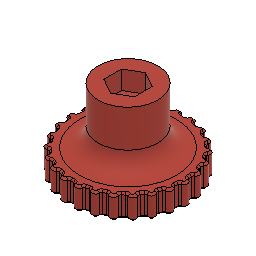
04 Laser Focus Knob v1 (Autodesk Fusion 360 design; units mm, degrees)
Autodesk Fusion 360 part; units mm, degrees
note: some values were not read from the file. Set by a fixed rule: which sketch regions a step uses.
sketch "Sketch1" plane through (0, 0, 0) normal (0, 1, 0) x (1, 0, 0)
  circle A0 centre (0, 0) radius 15
  dimension "d1" = 30
  constraint coincident A0.centre origin
  measures "d1" diameter of A0
extrude "Extrude1" add sketch "Sketch1" along normal blind 6
sketch "Sketch2" plane through (0, 6, 0) normal (0, 1, 0) x (-1, 0, 0)
  circle A0 centre (0, 0) radius 15
  circle A1 centre (0, 0) radius 8
  dimension "d4" = 16
  constraint concentric A0 A1
  measures "d4" diameter of A1
extrude "Extrude2" add sketch "Sketch2" along normal blind 15 contours A1
sketch "Sketch3" plane through (0, 21, 0) normal (0, 1, 0) x (-1, 0, 0)
  circle A0 centre (0, 0) radius 8
  circle A1 centre (0, 0) radius 2.625
  dimension "d7" = 5.25
  constraint concentric A0 A1
  measures "d7" diameter of A1
extrude "Extrude3" cut sketch "Sketch3" against normal blind 50 contours A1
sketch "Sketch4" plane through (0, 0, 0) normal (0, -1, 0) x (1, 0, 0)
  circle A0 centre (0, 0) radius 2.625
  circle A1 centre (0, 0) radius 15
  circle A2 centre (0, 0) radius 5
  dimension "d10" = 10
  constraint concentric A0 A2
  measures "d10" diameter of A2
extrude "Extrude4" cut sketch "Sketch4" against normal blind 12 contours A2
sketch "Sketch5" plane through (0, 21, 0) normal (0, 1, 0) x (-1, 0, 0)
  circle A0 centre (0, 0) radius 2.625
  circle A1 centre (0, 0) radius 8
  line L0 (-4.1, -2.3671) -> (0, -4.7343)
  line L1 (0, -4.7343) -> (4.1, -2.3671)
  line L2 (4.1, -2.3671) -> (4.1, 2.3671)
  line L3 (4.1, 2.3671) -> (0, 4.7343)
  line L4 (0, 4.7343) -> (-4.1, 2.3671)
  line L5 (-4.1, 2.3671) -> (-4.1, -2.3671)
  dimension "d27" = 8.2
  constraint coincident A0.centre A1.centre
  measures "d27" distance of L2 L5
extrude "Extrude5" cut sketch "Sketch5" against normal blind 5 contours L0 L1 L2 L3 L4 L5
sketch "Sketch6" plane through (0, 0, 0) normal (0, -1, 0) x (1, 0, 0)
  circle A0 centre (0, 0) radius 5
  circle A1 centre (0, 0) radius 15
  circle A2 centre (-15, 0) radius 1
  point P0 (-15, 0)
  dimension "d15" = 2
  constraint coincident P0 A2.centre
  measures "d15" diameter of A2
extrude "Extrude6" add sketch "Sketch6" against normal blind 6 contours A1 A2 | A1 A2 picked at (-14.6642, 0) picked at (-15.3309, 0)
fillet "Fillet1" radius 0.5 1 edges at (-14.9667, 3, 0.9994)
fillet "Fillet2" radius 0.5 1 edges at (-14.9667, 3, -0.9994)
pattern_circular "C-Pattern1" count 26 over 360 about axis through (0, 1.75, 0) along (0, 1, 0) of "Extrude6", "Fillet1", "Fillet2"
chamfer "Chamfer1" distance 0.5 angle 45 208 edges at (-9.089, 0, 13.1677) (-9.4686, 0, 11.7468) (-9.9468, 0, 11.2277) (-10.5198, 0, 10.8155) (-11.9762, 0, 10.61) (-12.0047, 0, 9.1394) (-12.3448, 0, 8.521) (-12.8024, 0, 7.9837) (-14.1673, 0, 7.4356) (-13.8431, 0, 6.001) (-14.0252, 0, 5.3191) (-14.341, 0, 4.6879) (-15.5351, 0, 3.8291) (-14.8769, 0, 2.5137) (-14.8906, 0, 1.8081) (-15.0462, 0, 1.1196) (-16, 0, 0) (-15.0462, 0, -1.1196) (-14.8906, 0, -1.8081) (-14.8769, 0, -2.5137) (-15.5351, 0, -3.8291) (-14.341, 0, -4.6879) (-14.0252, 0, -5.3191) (-13.8431, 0, -6.001) (-14.1673, 0, -7.4356) (-12.8024, 0, -7.9837) (-12.3448, 0, -8.521) (-12.0047, 0, -9.1394) (-11.9762, 0, -10.61) (-10.5198, 0, -10.8155) (-9.9468, 0, -11.2277) (-9.4686, 0, -11.7468) (-9.089, 0, -13.1677) (-7.6258, 0, -13.0188) (-6.9708, 0, -13.2818) (-6.3823, 0, -13.6714) (-5.6737, 0, -14.9603) (-4.2886, 0, -14.4655) (-3.5897, 0, -14.5641) (-2.9251, 0, -14.8015) (-1.9286, 0, -15.8833) (-0.7022, 0, -15.0715) (0, 0, -15) (0.7022, 0, -15.0715) (1.9286, 0, -15.8833) (2.9251, 0, -14.8015) (3.5897, 0, -14.5641) (4.2886, 0, -14.4655) (5.6737, 0, -14.9603) (6.3823, 0, -13.6714) (6.9708, 0, -13.2818) (7.6258, 0, -13.0188) (9.089, 0, -13.1677) (9.4686, 0, -11.7468) (9.9468, 0, -11.2277) (10.5198, 0, -10.8155) (11.9762, 0, -10.61) (12.0047, 0, -9.1394) (12.3448, 0, -8.521) (12.8024, 0, -7.9837) (14.1673, 0, -7.4356) (13.8431, 0, -6.001) (14.0252, 0, -5.3191) (14.341, 0, -4.6879) (15.5351, 0, -3.8291) (14.8769, 0, -2.5137) (14.8906, 0, -1.8081) (15.0462, 0, -1.1196) (16, 0, 0) (15.0462, 0, 1.1196) (14.8906, 0, 1.8081) (14.8769, 0, 2.5137) (15.5351, 0, 3.8291) (14.341, 0, 4.6879) (14.0252, 0, 5.3191) (13.8431, 0, 6.001) (14.1673, 0, 7.4356) (12.8024, 0, 7.9837) (12.3448, 0, 8.521) (12.0047, 0, 9.1394) (11.9762, 0, 10.61) (10.5198, 0, 10.8155) (9.9468, 0, 11.2277) (9.4686, 0, 11.7468) (9.089, 0, 13.1677) (7.6258, 0, 13.0188) (6.9708, 0, 13.2818) (6.3823, 0, 13.6714) (5.6737, 0, 14.9603) (4.2886, 0, 14.4655) (3.5897, 0, 14.5641) (2.9251, 0, 14.8015) (1.9286, 0, 15.8833) (0.7022, 0, 15.0715) (0, 0, 15) (-0.7022, 0, 15.0715) (-1.9286, 0, 15.8833) (-2.9251, 0, 14.8015) (-3.5897, 0, 14.5641) (-4.2886, 0, 14.4655) (-5.6737, 0, 14.9603) (-6.3823, 0, 13.6714) (-6.9708, 0, 13.2818) (-7.6258, 0, 13.0188) (-15.5351, 6, 3.8291) (-14.341, 6, 4.6879) (-14.0252, 6, 5.3191) (-13.8431, 6, 6.001) (-14.1673, 6, 7.4356) (-12.8024, 6, 7.9837) (-12.3448, 6, 8.521) (-12.0047, 6, 9.1394) (-11.9762, 6, 10.61) (-10.5198, 6, 10.8155) (-9.9468, 6, 11.2277) (-9.4686, 6, 11.7468) (-9.089, 6, 13.1677) (-7.6258, 6, 13.0188) (-6.9708, 6, 13.2818) (-6.3823, 6, 13.6714) (-5.6737, 6, 14.9603) (-4.2886, 6, 14.4655) (-3.5897, 6, 14.5641) (-2.9251, 6, 14.8015) (-1.9286, 6, 15.8833) (-0.7022, 6, 15.0715) (0, 6, 15) (0.7022, 6, 15.0715) (1.9286, 6, 15.8833) (2.9251, 6, 14.8015) (3.5897, 6, 14.5641) (4.2886, 6, 14.4655) (5.6737, 6, 14.9603) (6.3823, 6, 13.6714) (6.9708, 6, 13.2818) (7.6258, 6, 13.0188) (9.089, 6, 13.1677) (9.4686, 6, 11.7468) (9.9468, 6, 11.2277) (10.5198, 6, 10.8155) (11.9762, 6, 10.61) (12.0047, 6, 9.1394) (12.3448, 6, 8.521) (12.8024, 6, 7.9837) (14.1673, 6, 7.4356) (13.8431, 6, 6.001) (14.0252, 6, 5.3191) (14.341, 6, 4.6879) (15.5351, 6, 3.8291) (14.8769, 6, 2.5137) (14.8906, 6, 1.8081) (15.0462, 6, 1.1196) (16, 6, 0) (15.0462, 6, -1.1196) (14.8906, 6, -1.8081) (14.8769, 6, -2.5137) (15.5351, 6, -3.8291) (14.341, 6, -4.6879) (14.0252, 6, -5.3191) (13.8431, 6, -6.001) (14.1673, 6, -7.4356) (12.8024, 6, -7.9837) (12.3448, 6, -8.521) (12.0047, 6, -9.1394) (11.9762, 6, -10.61) (10.5198, 6, -10.8155) (9.9468, 6, -11.2277) (9.4686, 6, -11.7468) (9.089, 6, -13.1677) (7.6258, 6, -13.0188) (6.9708, 6, -13.2818) (6.3823, 6, -13.6714) (5.6737, 6, -14.9603) (4.2886, 6, -14.4655) (3.5897, 6, -14.5641) (2.9251, 6, -14.8015) (1.9286, 6, -15.8833) (0.7022, 6, -15.0715) (0, 6, -15) (-0.7022, 6, -15.0715) (-1.9286, 6, -15.8833) (-2.9251, 6, -14.8015) (-3.5897, 6, -14.5641) (-4.2886, 6, -14.4655) (-5.6737, 6, -14.9603) (-6.3823, 6, -13.6714) (-6.9708, 6, -13.2818) (-7.6258, 6, -13.0188) (-9.089, 6, -13.1677) (-9.4686, 6, -11.7468) (-9.9468, 6, -11.2277) (-10.5198, 6, -10.8155) (-11.9762, 6, -10.61) (-12.0047, 6, -9.1394) (-12.3448, 6, -8.521) (-12.8024, 6, -7.9837) (-14.1673, 6, -7.4356) (-13.8431, 6, -6.001) (-14.0252, 6, -5.3191) (-14.341, 6, -4.6879) (-15.5351, 6, -3.8291) (-14.8769, 6, -2.5137) (-14.8906, 6, -1.8081) (-15.0462, 6, -1.1196) (-16, 6, 0) (-15.0462, 6, 1.1196) (-14.8906, 6, 1.8081) (-14.8769, 6, 2.5137)
fillet "Fillet3" radius 5 1 edges at (7.4586, 6, 2.8929)
sketch "Sketch7" plane through (0, 0, 0) normal (0, 1, 0) x (-1, 0, 0)
